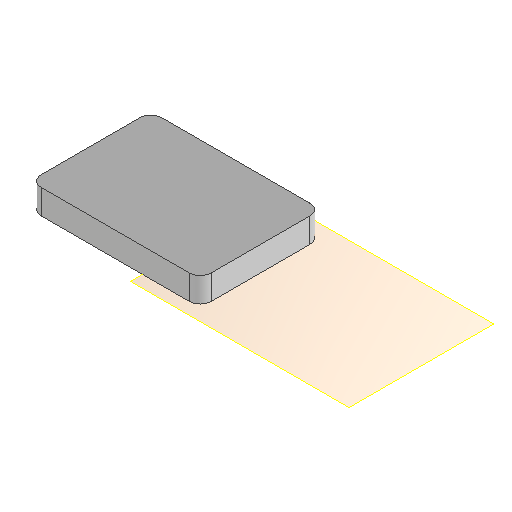
# Autodesk Inventor part: 20_Cube_4_insert_Lens_kinematic_mirrormount_plate
Saved by Autodesk Inventor 2025.1 (Build 291241020, 241B)
## iProperties
Created: 2024-10-03
Part Number: 20_Cube_4_insert_Lens_kinematic_mirrormount_plate
Material: Generic
Document SubType Name: Modeling
Designer: diederichbenedict
Density: 1 g/cm^3
Appearance: Default
Author: diederichbenedict
Autodesk Inventor part; units mm, degrees
ref_plane "YZ Plane" through (0, 0, 0) normal (1, 0, 0) x (0, 1, 0)
ref_plane "XZ Plane" through (0, 0, 0) normal (0, 1, 0) x (-1, 0, 0)
ref_plane "XY Plane" through (0, 0, 0) normal (0, 0, 1) x (1, 0, 0)
ref_plane "Work Plane1" through (24.9, 0, 1) normal (0, 0, 1) x (1, 0, 0)
sketch "Sketch1" plane through (24.9, 0, 1) normal (0, 0, 1) x (1, 0, 0)
  circle A0 centre (-55.5143, -4) radius 2.45
  circle A1 centre (-30.5143, -4) radius 2.45
  circle A2 centre (-30.5143, -20) radius 2.45
  line L0 (-55.5143, -4) -> (-30.5143, -4)
  line L1 (-30.5143, -4) -> (-30.5143, -20)
  line L2 (-30.5143, -20) -> (-55.5143, -20)
  line L3 (-55.5143, -20) -> (-55.5143, -4)
  line L4 (-27.5143, -1) -> (-58.5143, -1)
  line L5 (-58.5143, -1) -> (-58.5143, -23)
  line L6 (-58.5143, -23) -> (-27.5143, -23)
  line L7 (-27.5143, -23) -> (-27.5143, -1)
  circle A3 centre (-55.5143, -4) radius 1.4 projected
  circle A4 centre (-30.5143, -4) radius 1.4 projected
  circle A5 centre (-30.5143, -20) radius 1.4 projected
  circle A6 centre (-55.5143, -20) radius 1.4 projected
  dimension "d0" = 4.9
  dimension "d1" = 4.9
  dimension "d2" = 4.9
  dimension "d3" = 3
  constraints: 16 end point, 4 parallel, 3 centre point, 3 coincident, 2 perpendicular, 1 horizontal, 3 other
  measures "d0" diameter of A0
  measures "d1" diameter of A1
  measures "d2" diameter of A2
  measures "d3" distance between parallel lines of L0 L4
extrude "Extrusion1" add sketch "Sketch1" along normal blind 3.5 contours L0 A1 L1 A2 L2 A6 L3 A0 | L7 L6 L5 L4
sketch "Sketch2" plane through (24.9, 0, 4.5) normal (0, 0, 1) x (1, 0, 0)
  circle A0 centre (-30.5143, -4) radius 2.45 projected
  circle A1 centre (-30.5143, -20) radius 2.45 projected
  circle A2 centre (-55.5143, -4) radius 2.45 projected
  line L0 (-58.5143, -1) -> (-58.5143, -23) projected
  line L1 (-58.5143, -23) -> (-27.5143, -23) projected
  line L2 (-27.5143, -23) -> (-27.5143, -1) projected
  line L3 (-27.5143, -1) -> (-58.5143, -1) projected
  circle A3 centre (-55.5143, -20) radius 1.4 projected
  circle A4 centre (-30.5143, -20) radius 2.45 projected
  circle A5 centre (-30.5143, -4) radius 2.45 projected
  circle A6 centre (-55.5143, -4) radius 2.45 projected
  point P0 (-24.9, 0)
extrude "Extrusion2" add sketch "Sketch2" along normal blind 1 contours A0 | A1 | A2 | L3 L2 L1 L0 | A3
fillet "Fillet1" radius 2 4 edges at (-33.6143, -23, 3.25) (-2.6143, -23, 3.25) (-33.6143, -1, 3.25) (-2.6143, -1, 3.25)
equation "\"d1\" = d0"
equation "\"d2\" = d0"
body "Solid1"
